Autodesk Fusion 360 part; units mm, degrees
(part 2 of 2)
  constraint concentric A23 A144
  constraint concentric A22 A145
  constraint concentric A21 A146
  constraint concentric A20 A147
  constraint concentric A19 A148
  constraint concentric A18 A149
  constraint concentric A16 A151
  constraint concentric A15 A152
  constraint concentric A14 A153
  constraint concentric A13 A154
  constraint tangent A134 L135
  constraint tangent A133 L134
  constraint tangent A136 L137
  constraint tangent L133 A154
  constraint tangent L134 A134
  constraint tangent A146 L147
  constraint tangent A135 L136
  constraint tangent A152 L153
  constraint tangent A137 L138
  constraint tangent A138 L139
  constraint tangent A139 L140
  constraint tangent A140 L141
  constraint tangent L141 A141
  constraint tangent A145 L146
  constraint tangent A142 L143
  constraint tangent L143 A143
  constraint tangent A143 L144
  constraint tangent A144 L145
  constraint tangent A148 L149
  constraint tangent A147 L148
  constraint tangent A149 L150
  constraint tangent A150 L151
  constraint tangent A151 L152
  constraint tangent A153 L154
  constraint tangent A246 L245
  constraint tangent L246 A251
  constraint tangent L246 A252
  constraint tangent L247 A253
  constraint tangent L247 A254
  constraint tangent L237 A255
  constraint tangent L238 A255
  constraint tangent L235 A256
  constraint tangent L236 A256
  constraint tangent L241 A257
  constraint tangent L242 A257
  constraint tangent L226 A258
  constraint tangent L227 A258
  constraint tangent L229 A259
  constraint tangent L230 A259
  constraint tangent L231 A260
  constraint tangent L232 A260
  constraint coincident L142 L248.start
  constraint coincident L232 L248.end
  constraint perpendicular L232 L248
  constraint coincident L143 L249.start
  constraint coincident L233 L249.end
  constraint perpendicular L233 L249
  constraint tangent A250 L250
  constraint tangent A238 L251
  constraint tangent L250 A261
  constraint tangent L251 A261
  constraint tangent L243 A262
  constraint tangent L244 A262
  constraint tangent L244 A263
  constraint tangent L245 A263
  measures "d1" diameter of A0
  measures "d2" diameter of A1
  measures "d3" diameter of A2
  measures "d4" diameter of A3
  measures "d5" diameter of A4
  measures "d9" diameter of A110
  measures "d12" diameter of A111
  measures "d318" diameter of A159
  measures "d319" diameter of A160
extrude "Extrude1" add sketch "mriya-bumper-mjf" along normal blind 10.5 contours L133 A133 L134 A134 L135 A135 L136 A136 L137 A137 L138 A138 L139 A139 L140 A140 L141 A141 L142 L143 A143 L144 A144 L145 A145 L146 A146 L147 A147 L148 A148 L149 A149 L150 A150 L151 A151 L152 A152 L153 A153 L154 A154 A238 L226 L227 A239 L228 A240 L229 L230 A241 L231 L232 L233 A243 L234 A244 L235 L236 A245 L237 L238 A246 A247 L239 A248 L240 A249 L241 L242 A250 L243 L244 L245 A255 A256 A257 A258 A259 A260 L248 L249 L250 L251 A261 A262 A263 makes body 1
extrude "Extrude2" add sketch "mriya-bumper-mjf" along normal blind 17 contours L142 A142 L143 L232 A242 L233 L248 L249 bodies 1
extrude "Extrude3" add sketch "mriya-bumper-mjf" along normal blind 2 from surface at 1.7 contours A113 | A114 | A115 | A116 | L133 A133 L134 A134 L135 A135 L136 A136 L137 A137 L138 A138 L139 A139 L140 A140 L141 A141 L142 A142 L143 A143 L144 A144 L145 A145 L146 A146 L147 A147 L148 A148 L149 A149 L150 A150 L151 A151 L152 A152 L153 A153 L154 A154 L246 A251 A252 L247 A253 A254 | L142 L246 A251 A252 | L143 L247 A253 A254 | A159 | A160 bodies 1
extrude "Extrude6" add sketch "mriya-bumper-mjf" along normal blind 1 from surface at 14.3 contours L142 L246 A251 A252 bodies 1
extrude "Extrude13" add sketch "mriya-bumper-mjf" along normal blind 1 from surface at 7.7 contours L143 L247 A253 A254 bodies 1
extrude "Extrude14" cut sketch "mriya-bumper-mjf" along normal blind 2.7 contours A159 | A160 bodies 1
chamfer "Chamfer10" distance 0.7 angle 45 2 edges at (-16.4, 78.0932, 14.3) (-7, 9.5932, 7.7) on bodies 1
sketch "power-switch" plane through (-4.4, 0, 0) normal (1, 0, 0) x (0, 1, 0)
  line L0 (35.9932, 5.4) -> (25.7932, 5.4)
  line L1 (25.7932, 5.4) -> (25.7932, 8.1)
  line L2 (25.7932, 8.1) -> (35.9932, 8.1)
  line L3 (35.9932, 8.1) -> (35.9932, 5.4)
  line L4 (36.3932, 4) -> (25.3932, 4)
  line L5 (24.3932, 5) -> (24.3932, 8.5)
  line L6 (25.3932, 9.5) -> (36.3932, 9.5)
  line L7 (37.3932, 8.5) -> (37.3932, 5)
  arc A0 (25.3932, 9.5) -> (24.3932, 8.5) centre (25.3932, 8.5) ccw
  arc A1 (37.3932, 8.5) -> (36.3932, 9.5) centre (36.3932, 8.5) ccw
  arc A2 (24.3932, 5) -> (25.3932, 4) centre (25.3932, 5) ccw
  arc A3 (36.3932, 4) -> (37.3932, 5) centre (36.3932, 5) ccw
  line L8 (1.9932, 0) -> (76.4932, 0)
  line L9 (76.4932, 0) -> (76.4932, 17)
  line L10 (76.4932, 17) -> (19.3955, 17)
  line L11 (19.3955, 17) -> (19.3955, 10.5)
  line L12 (19.3955, 10.5) -> (1.9932, 10.5)
  line L13 (1.9932, 10.5) -> (1.9932, 0)
  constraint perpendicular L0 L1
  constraint vertical L1
  constraint perpendicular L1 L2
  constraint vertical L3
  constraint tangent L6 A0
  constraint tangent L5 A0
  constraint tangent L7 A1
  constraint tangent L6 A1
  constraint tangent L5 A2
  constraint tangent L4 A2
  constraint tangent L4 A3
  constraint tangent L7 A3
extrude "Extrude8" cut sketch "power-switch" against normal blind 2.6 contours L0 L1 L2 L3 bodies 1
extrude "Extrude9" cut sketch "power-switch" against normal blind 1.2 contours L4 L5 L6 L7 A0 A1 A2 A3 bodies 1
chamfer "Chamfer11" distance 1.2 angle 45 8 edges at (-4.4, 30.8932, 9.5) (-4.4, 37.1003, 9.2071) (-4.4, 37.3932, 6.75) (-4.4, 37.1003, 4.2929) (-4.4, 30.8932, 4) (-4.4, 24.6861, 4.2929) (-4.4, 24.3932, 6.75) (-4.4, 24.6861, 9.2071) on bodies 1
chamfer "Chamfer13" distance 0.4 angle 45 1 edges at (-7, 30.8932, 8.1) on bodies 1
sketch "usb-c" plane through (0, 80.6932, 0) normal (0, 1, 0) x (-1, 0, 0)
  line L0 (19.7003, 7.95) -> (13.1002, 7.95)
  line L1 (13.1002, 12.35) -> (19.7002, 12.35)
  line L2 (19.7002, 8.85) -> (13.1002, 8.85)
  line L3 (21.0002, 11.05) -> (21.0002, 10.15)
  line L4 (13.1002, 13.25) -> (19.7002, 13.25)
  line L5 (11.8003, 10.15) -> (11.8003, 11.05)
  arc A0 (13.1002, 12.35) -> (11.8003, 11.05) centre (13.1002, 11.05) ccw
  arc A1 (11.8003, 10.15) -> (13.1003, 8.85) centre (13.1002, 10.15) ccw
  arc A2 (21.0002, 11.05) -> (19.7002, 12.35) centre (19.7002, 11.05) ccw
  arc A3 (19.7002, 8.85) -> (21.0002, 10.15) centre (19.7003, 10.15) ccw
  line L6 (21.9002, 11.05) -> (21.9002, 10.15)
  line L7 (10.9002, 11.05) -> (10.9002, 10.15)
  arc A4 (21.9002, 11.05) -> (19.7003, 13.25) centre (19.7003, 11.05) ccw
  arc A5 (19.7003, 7.95) -> (21.9002, 10.15) centre (19.7002, 10.15) ccw
  arc A6 (13.1002, 13.25) -> (10.9002, 11.05) centre (13.1002, 11.05) ccw
  arc A7 (10.9002, 10.15) -> (13.1002, 7.95) centre (13.1002, 10.15) ccw
  line L8 (8.6, 0) -> (40.8603, 0)
  line L9 (40.8603, 0) -> (40.8603, 10.5)
  line L10 (40.8603, 10.5) -> (25.7, 10.5)
  line L11 (25.7, 10.5) -> (25.7, 17)
  line L12 (25.7, 17) -> (8.6, 17)
  line L13 (8.6, 17) -> (8.6, 0)
  constraint horizontal L0
  constraint tangent L5 A0
  constraint tangent L1 A0
  constraint tangent L2 A1
  constraint tangent L5 A1
  constraint tangent L1 A2
  constraint tangent L3 A2
  constraint tangent L3 A3
  constraint tangent L2 A3
  constraint parallel L5 L6
  constraint tangent L6 A4
  constraint tangent L4 A4
  constraint tangent L0 A5
  constraint tangent L6 A5
  constraint tangent L4 A6
  constraint tangent L7 A6
  constraint tangent L7 A7
  constraint tangent L0 A7
extrude "Extrude10" cut sketch "usb-c" against normal blind 2.6 contours L1 L2 L3 L5 A0 A1 A2 A3 bodies 1
extrude "Extrude11" cut sketch "usb-c" against normal blind 1.2 contours L0 L4 L6 L7 A4 A5 A6 A7 bodies 1
chamfer "Chamfer12" distance 1.2 angle 45 8 edges at (-16.4003, 80.6932, 7.95) (-11.5446, 80.6932, 8.5944) (-10.9003, 80.6932, 10.6) (-11.5446, 80.6932, 12.6056) (-16.4003, 80.6932, 13.25) (-21.2559, 80.6932, 12.6056) (-21.9003, 80.6932, 10.6) (-21.2559, 80.6932, 8.5944) on bodies 1
fillet "Fillet31" radius 1.6 90 edges at (-4.4, 47.9443, 17) (-5.6302, 79.463, 17) (-17.15, 80.6932, 17) (-33.2802, 80.6932, 10.5) (-41.4343, 80.8074, 10.5) (-42.163, 81.3746, 10.5) (-43.9298, 82.6354, 10.5) (-51.6943, 82.9932, 10.5) (-58.2343, 83.1074, 10.5) (-60.063, 84.7746, 10.5) (-62.9298, 87.1354, 10.5) (-73.4, 87.4932, 10.5) (-83.8702, 87.1354, 10.5) (-86.237, 85.2746, 10.5) (-87.5657, 84.1074, 10.5) (-94.6056, 83.9932, 10.5) (-102.8702, 83.6354, 10.5) (-107.4138, 79.5978, 10.5) (-111.0814, 76.1454, 10.5) (-115.9592, 75.9932, 10.5) (-121.8702, 75.6354, 10.5) (-123.637, 74.3746, 10.5) (-124.3657, 73.8074, 10.5) (-131.5198, 73.6932, 10.5) (-141.0698, 72.463, 10.5) (-142.3, 42.8932, 10.5) (-141.0698, 13.3234, 10.5) (-120.6213, 12.0932, 10.5) (-100.9613, 12.5271, 10.5) (-96.2397, 16.6351, 10.5) (-92.7186, 19.941, 10.5) (-84.5898, 20.0932, 10.5) (-75.7143, 19.6842, 10.5) (-70.7197, 11.6751, 10.5) (-65.1018, 3.0339, 10.5) (-55.8362, 2.3932, 10.5) (-48.3657, 2.279, 10.5) (-47.637, 1.7118, 10.5) (-45.8702, 0.451, 10.5) (-37.0056, 0.0932, 10.5) (-29.3657, -0.021, 10.5) (-28.637, -0.5882, 10.5) (-26.8702, -1.849, 10.5) (-16.8358, -2.2068, 10.5) (-5.6302, -0.9766, 10.5) (-4.4, 10.6943, 10.5) (-5.6302, 79.463, 0) (-4.4, 39.2432, 0) (-5.6302, -0.9766, 0) (-16.8358, -2.2068, 0) (-26.8702, -1.849, 0) (-28.637, -0.5882, 0) (-29.3657, -0.021, 0) (-37.0056, 0.0932, 0) (-45.8702, 0.451, 0) (-47.637, 1.7118, 0) (-48.3657, 2.279, 0) (-55.8362, 2.3932, 0) (-65.1018, 3.0339, 0) (-70.7197, 11.6751, 0) (-75.7143, 19.6842, 0) (-84.5898, 20.0932, 0) (-92.7186, 19.941, 0) (-96.2397, 16.6351, 0) (-100.9613, 12.5271, 0) (-120.6213, 12.0932, 0) (-141.0698, 13.3234, 0) (-142.3, 42.8932, 0) (-141.0698, 72.463, 0) (-131.5198, 73.6932, 0) (-124.3657, 73.8074, 0) (-123.637, 74.3746, 0) (-121.8702, 75.6354, 0) (-115.9592, 75.9932, 0) (-111.0814, 76.1454, 0) (-107.4138, 79.5978, 0) (-102.8702, 83.6354, 0) (-94.6056, 83.9932, 0) (-87.5657, 84.1074, 0) (-86.237, 85.2746, 0) (-83.8702, 87.1354, 0) (-73.4, 87.4932, 0) (-62.9298, 87.1354, 0) (-60.063, 84.7746, 0) (-58.2343, 83.1074, 0) (-51.6943, 82.9932, 0) (-43.9298, 82.6354, 0) (-42.163, 81.3746, 0) (-41.4343, 80.8074, 0) (-24.7302, 80.6932, 0) on bodies 1
fillet "Fillet32" radius 0.6 6 edges at (-25.7, 80.6932, 12.15) (-25.7, 80.2246, 16.5314) (-25.7, 78.5932, 17) (-4.4, 19.3955, 12.15) (-4.8686, 19.3955, 16.5314) (-6.5, 19.3955, 17) on bodies 1
mirror "Mirror1" about plane through (0, 0, 0) normal (1, 0, 0) of bodies 1 makes body 2
named bodies: "Left", "Right"
